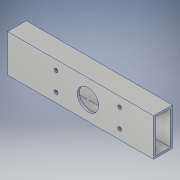
# Autodesk Inventor part: gearboxsupportbar
Saved by Autodesk Inventor 2019 (Build 230136000, 136)
## iProperties
Created: 2019-01-13
Part Number: gearboxsupportbar
Material: Aluminum 6061
Document SubType Name: Modeling
Designer: lebraddock
Density: 2.7 g/cm^3
Appearance: Aluminum - Flat
Author: lebraddock
Autodesk Inventor part; units mm, degrees
ref_plane "YZ Plane" through (0, 0, 0) normal (1, 0, 0) x (0, 1, 0)
ref_plane "XZ Plane" through (0, 0, 0) normal (0, 1, 0) x (-1, 0, 0)
ref_plane "XY Plane" through (0, 0, 0) normal (0, 0, 1) x (1, 0, 0)
sketch "Sketch1" plane through (0, 0, 0) normal (0, 0, 1) x (1, 0, 0)
  circle A0 centre (0, 0) radius 14.2875
  line L0 (88.4644, 25.4) -> (-108.3818, 25.4)
  line L1 (-108.3818, 25.4) -> (-108.3818, -25.4)
  line L2 (-108.3818, -25.4) -> (88.4644, -25.4)
  line L3 (88.4644, -25.4) -> (88.4644, 25.4)
  dimension "d0" = 28.575
  dimension "d4" = 50.8
  dimension "d15" = 88.4644
  dimension "d16" = 108.3818
  constraints: 8 end point, 2 parallel, 1 centre point, 1 coincident, 1 horizontal, 1 perpendicular
  measures "d0" diameter of A0
  measures "d4" distance of L1.end L0.end
  measures "d15" distance from line of L3 point (0, 0)
  measures "d16" distance from line of L1 point (0, 0)
extrude "Extrusion1" add sketch "Sketch1" along normal blind 25.4
sketch "Sketch2" plane through (88.4644, -25.4, 0) normal (1, 0, 0) x (0, 0, -1)
  line L0 (0, 50.8) -> (-25.4, 50.8) projected
  line L1 (0, 0) -> (-25.4, 0) projected
  line L2 (0, 50.8) -> (-25.4, 50.8)
  line L3 (-25.4, 50.8) -> (-25.4, 0)
  line L4 (-25.4, 0) -> (0, 0)
  line L5 (0, 0) -> (0, 50.8)
  line L6 (-22.5778, 2.8222) -> (-22.5778, 47.9778)
  line L7 (-22.5778, 47.9778) -> (-2.8222, 47.9778)
  line L8 (-2.8222, 47.9778) -> (-2.8222, 2.8222)
  line L9 (-2.8222, 2.8222) -> (-22.5778, 2.8222)
  point P0 (0, 25.4)
  dimension "d7" = 2.8222
  constraints: 16 end point, 4 parallel, 2 perpendicular, 1 horizontal, 3 other
  measures "d7" distance between parallel lines of L3 L6
extrude "Extrusion2" cut sketch "Sketch2" against normal blind 203.2 contours L6 L7 L8 L9
sketch "Sketch3" plane through (0, 0, 25.4) normal (0, 0, 1) x (1, 0, 0)
  circle A0 centre (42.8752, 12.7) radius 2.5527
  circle A1 centre (42.8752, -12.7) radius 2.5527
  circle A2 centre (-42.8752, 12.7) radius 2.5527
  circle A3 centre (-42.8752, -12.7) radius 2.5527
  point P0 (0, 0)
  dimension "d12" = 5.1054
  constraints: 4 centre point
  measures "d12" diameter of A0
extrude "Extrusion3" cut sketch "Sketch3" against normal blind 25.4
sketch "Sketch4" plane through (0, 0, 25.4) normal (0, 0, 1) x (1, 0, 0)
  point P0 (0, 0)
body "Solid1"
